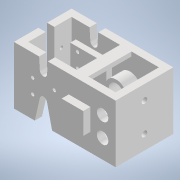
# Autodesk Inventor part: NewCasing
Saved by Autodesk Inventor 2020.1 (Build 241239000, 239)
## iProperties
Created: 2019-11-05
Part Number: NewCasing
Material: Generic
Document SubType Name: Modeling
Designer: ajtan
Density: 1 g/cm^3
Appearance: Default
Author: ajtan
Autodesk Inventor part; units mm, degrees
ref_plane "YZ Plane" through (0, 0, 0) normal (1, 0, 0) x (0, 1, 0)
ref_plane "XZ Plane" through (0, 0, 0) normal (0, 1, 0) x (-1, 0, 0)
ref_plane "XY Plane" through (0, 0, 0) normal (0, 0, 1) x (1, 0, 0)
sketch "Sketch1" plane through (0, 0, 0) normal (0, 0, 1) x (1, 0, 0)
  line L0 (-57.8485, 25.4) -> (-51.4985, 25.4)
  line L1 (-51.4985, 25.4) -> (-51.4985, -25.4)
  line L2 (-51.4985, -25.4) -> (-57.8485, -25.4)
  line L3 (-57.8485, -25.4) -> (-57.8485, 25.4)
  line L4 (25.4, 25.4) -> (31.75, 25.4)
  line L5 (31.75, 25.4) -> (31.75, -25.4)
  line L6 (31.75, -25.4) -> (25.4, -25.4)
  line L7 (25.4, -25.4) -> (25.4, 25.4)
  point P0 (0, 0)
  dimension "d0" = 6.35
  dimension "d1" = 50.8
  dimension "d2" = 25.4
  dimension "d3" = 51.4985
  dimension "d4" = 25.4
  dimension "d5" = 25.4
  constraints: 16 end point, 4 parallel, 2 equal length, 2 horizontal, 2 perpendicular
  measures "d0" distance of L1.end L2.end
  measures "d1" distance of L0.end L1.end
  measures "d2" distance from line of point (0, 0) L0
  measures "d3" distance from line of point (0, 0) L1
  measures "d4" distance from line of point (0, 0) L4
  measures "d5" distance from line of point (0, 0) L7
extrude "Extrusion1" add sketch "Sketch1" along normal mid plane 38.1
sketch "Sketch2" plane through (0, 0, 19.05) normal (0, 0, 1) x (1, 0, 0)
  line L0 (-51.4985, 25.4) -> (-57.8485, 25.4) projected
  line L1 (31.75, -25.4) -> (25.4, -25.4) projected
  line L2 (-57.8485, 25.4) -> (31.75, 25.4)
  line L3 (31.75, 25.4) -> (31.75, -25.4)
  line L4 (31.75, -25.4) -> (-57.8485, -25.4)
  line L5 (-57.8485, -25.4) -> (-57.8485, 25.4)
  circle A0 centre (0, 0) radius 6.604
  circle A1 centre (-41.3385, 6.35) radius 1.4605
  line L6 (-47.9108, 0) -> (-31.2118, 0) construction
  circle A2 centre (-41.3385, -6.35) radius 1.4605
  line L7 (-51.4985, -25.4) -> (-51.4985, 25.4) projected
  dimension "d8" = 13.208
  dimension "d40" = 2.921
  dimension "d42" = 19.05
  dimension "d43" = 16.51
  dimension "d44" = 6.35
  dimension "d92" = 6.35
  constraints: 10 end point, 3 centre point, 2 horizontal, 2 parallel, 1 coincident, 1 perpendicular, 1 symmetric about line, 1 other
  measures "d8" diameter of A0
  measures "d40" diameter of A1
  measures "d42" distance from line of L2 A1.centre
  measures "d43" distance from line of L5 A1.centre
  measures "d44" vertical distance of point (0, 0) A2.centre
  measures "d92" distance between parallel lines of L5 L7
sketch "Sketch3" plane through (0, 0, -19.05) normal (0, 0, -1) x (-1, 0, 0)
  line L0 (-31.75, 25.4) -> (-31.75, -25.4) projected
  line L1 (51.4985, -25.4) -> (57.8485, -25.4) projected
  line L2 (-31.75, 25.4) -> (57.8485, 25.4)
  line L3 (57.8485, 25.4) -> (57.8485, -25.4)
  line L4 (57.8485, -25.4) -> (-31.75, -25.4)
  line L5 (-31.75, -25.4) -> (-31.75, 25.4)
  circle A0 centre (0, 0) radius 6.604
  circle A1 centre (-11.43, 0.0226) radius 2.54
  circle A2 centre (-20.2438, 8.7122) radius 1.7907
  line L6 (-13.9699, 0) -> (6.604, 0) construction
  circle A3 centre (-20.2438, -8.7122) radius 1.7907
  circle A4 centre (41.3385, 6.35) radius 1.4605
  line L7 (51.4985, 25.4) -> (51.4985, -25.4) projected
  circle A5 centre (41.3385, -6.35) radius 1.4605
  dimension "d11" = 13.208
  dimension "d12" = 5.08
  dimension "d13" = 11.43
  dimension "d14" = 3.5814
  dimension "d15" = 20.2438
  dimension "d16" = 8.7122
  dimension "d32" = 2.921
  dimension "d33" = 10.16
  dimension "d34" = 6.35
  dimension "d35" = 6.35
  constraints: 10 end point, 4 centre point, 2 horizontal, 2 parallel, 2 symmetric about line, 1 coincident, 1 horizontal alignment, 1 perpendicular, 7 other
  measures "d13" distance of point (0, 0) point (-11.43, 0.023)
  measures "d14" diameter of A2
  measures "d15" horizontal distance of point (0, 0) A2.centre
  measures "d16" vertical distance of point (0, 0) A2.centre
  measures "d32" diameter of A4
  measures "d33" distance from line of A4.centre L7
  measures "d34" vertical distance of point (0, 0) A4.centre
  measures "d35" vertical distance of point (0, 0) A5.centre
extrude "Extrusion7" add sketch "Sketch2" along normal blind 6.35
extrude "Extrusion6" add sketch "Sketch3" along normal blind 6.35
sketch "Sketch6" plane through (-57.8485, -25.4, 25.4) normal (-1, 0, 0) x (0, 0, 1)
  circle A0 centre (-23.114, 38.1) radius 1.4605
  line L0 (-35.0625, 25.4) -> (-10.5897, 25.4) construction
  line L1 (0, 0) -> (-50.8, 0) construction
  line L2 (0, 50.8) -> (0, 0) construction
  circle A1 centre (-23.114, 12.7) radius 1.4605
  point P0 (-25.4, 25.4)
  dimension "d47" = 2.921
  dimension "d48" = 25.4
  dimension "d49" = 12.7
  dimension "d50" = 23.114
  constraints: 2 centre point, 2 end point, 1 horizontal, 1 symmetric about line, 1 other
  measures "d47" diameter of A0
  measures "d48" distance between parallel lines of L1 L0
  measures "d49" distance from line of L0 A0.centre
  measures "d50" distance from line of L2 A0.centre
extrude "Extrusion8" cut sketch "Sketch6" against normal up to next
sketch "Sketch8" plane through (-57.8485, 25.4, 25.4) normal (0, 1, 0) x (1, 0, 0)
  line L0 (0, 50.8) -> (0, 0) projected
  line L1 (0, 21.59) -> (6.35, 21.59)
  line L2 (6.35, 21.59) -> (6.35, 29.21)
  line L3 (6.35, 29.21) -> (0, 29.21)
  line L4 (0, 29.21) -> (0, 21.59)
  line L5 (0, 25.4) -> (6.35, 25.4) construction
  line L6 (89.5985, 0) -> (0, 0) projected
  line L7 (0, 50.8) -> (89.5985, 50.8) projected
  line L8 (6.35, 6.35) -> (6.35, 44.45) projected
  point P0 (57.8485, 25.4)
  point P1 (0, 29.21)
  dimension "d56" = 25.4
  dimension "d57" = 50.8
  dimension "d58" = 7.62
  constraints: 10 end point, 2 midpoint, 2 parallel, 1 collinear, 1 horizontal, 1 perpendicular, 1 point on line
  measures "d56" distance between parallel lines of L6 L5
  measures "d57" distance between parallel lines of L7 L6
  measures "d58" distance of L1.end L2.end
extrude "Extrusion10" cut sketch "Sketch8" against normal through all
sketch "Sketch10" plane through (0, 0, 25.4) normal (0, 0, 1) x (1, 0, 0)
  circle A0 centre (20.2438, -8.7122) radius 1.7907 construction
  circle A1 centre (20.2438, -8.7122) radius 1.7907 projected
  circle A2 centre (20.2438, 8.7122) radius 1.7907 construction
  circle A3 centre (20.2438, 8.7122) radius 1.7907 projected
  circle A4 centre (20.2438, 8.7122) radius 5.08
  circle A5 centre (20.2438, -8.7122) radius 5.08
  point P0 (0, 0)
  dimension "d64" = 10.16
  constraints: 2 centre point, 2 coincident, 1 equal radius
  measures "d64" diameter of A4
extrude "Extrusion12" cut sketch "Sketch10" against normal blind 25.4 contours A1 | A3 | A4 | A5
sketch "Sketch11" plane through (0, 0, 25.4) normal (0, 0, 1) x (1, 0, 0)
  line L0 (9.525, -9.525) -> (-9.525, -9.525)
  line L1 (-9.525, -9.525) -> (-9.525, 9.525)
  line L2 (-9.525, 9.525) -> (9.525, 9.525)
  line L3 (9.525, 9.525) -> (9.525, -9.525)
  line L4 (9.525, -9.525) -> (-9.525, 9.525) construction
  line L5 (-9.525, -9.525) -> (9.525, 9.525) construction
  point P0 (0, 0)
  dimension "d67" = 19.05
  dimension "d68" = 19.05
  constraints: 12 end point, 2 midpoint, 2 parallel, 1 horizontal, 1 perpendicular
  measures "d67" distance of L1.end L2.end
  measures "d68" distance of L2.end L0.start
extrude "Extrusion13" add sketch "Sketch11" along normal blind 6.35
sketch "Sketch12" plane through (0, 0, -25.4) normal (0, 0, -1) x (-1, 0, 0)
  circle A0 centre (31.8389, -6.35) radius 3.175
  line L0 (57.8485, -25.4) -> (57.8485, 25.4) projected
  line L1 (34.9338, -5.6412) -> (39.4589, -25.4)
  line L2 (28.744, -5.6412) -> (24.2189, -25.4)
  line L3 (24.2189, -25.4) -> (39.4589, -25.4)
  line L4 (-25.4, -25.4) -> (51.4985, -25.4) projected
  circle A1 centre (31.8389, 15.24) radius 3.175
  line L5 (57.8485, 25.4) -> (-31.75, 25.4) projected
  line L6 (28.67, 15.0438) -> (28.0289, 25.4)
  line L7 (51.4985, 25.4) -> (-25.4, 25.4) projected
  line L8 (35.0078, 15.0438) -> (35.6489, 25.4)
  point P0 (0, 0)
  dimension "d71" = 6.35
  dimension "d72" = 26.0096
  dimension "d73" = 6.35
  dimension "d74" = 15.24
  dimension "d75" = 7.62
  dimension "d78" = 10.16
  dimension "d79" = 7.62
  dimension "d80" = 3.81
  constraints: 10 end point, 4 point on circle, 4 tangent, 2 centre point, 2 collinear, 2 point on line, 1 equal radius, 1 vertical alignment
  measures "d71" vertical distance of point (0, 0) A0.centre
  measures "d72" distance from line of L0 A0.centre
  measures "d73" diameter of A0
  measures "d74" distance of L2.end L1.end
  measures "d75" horizontal distance of L2.end A0.centre
  measures "d78" distance from line of L5 A1.centre
  measures "d79" distance of L8.end L6.end
  measures "d80" horizontal distance of A1.centre L6.end
extrude "Extrusion14" cut sketch "Sketch12" against normal through all
sketch "Sketch13" plane through (0, 0, -19.05) normal (0, 0, 1) x (1, 0, 0)
  circle A0 centre (0, 0) radius 6.604 projected
  circle A1 centre (0, 0) radius 6.604 projected
  circle A2 centre (0, 0) radius 9.525
  dimension "d81" = 19.05
  constraints: 1 centre point, 1 coincident
  measures "d81" diameter of A2
extrude "Extrusion15" add sketch "Sketch13" along normal blind 12.192
sketch "Sketch14" plane through (31.75, 25.4, 25.4) normal (0, 1, 0) x (1, 0, 0)
  line L0 (-59.7789, 50.8) -> (0, 50.8) projected
  line L1 (-22.225, 0) -> (-41.275, 0) projected
  line L2 (-40.64, 50.8) -> (-30.48, 50.8)
  line L3 (-30.48, 50.8) -> (-30.48, 0)
  line L4 (-30.48, 0) -> (-40.64, 0)
  line L5 (-40.64, 0) -> (-40.64, 50.8)
  line L6 (0, 0) -> (0, 50.8) projected
  point P0 (-31.75, 25.4)
  dimension "d84" = 10.16
  dimension "d85" = 40.64
  constraints: 8 end point, 2 parallel, 2 point on line, 1 horizontal, 1 perpendicular
  measures "d84" distance between parallel lines of L5 L3
  measures "d85" distance between parallel lines of L6 L5
extrude "Extrusion16" add sketch "Sketch14" against normal blind 3.81
sketch "Sketch15" plane through (0, 0, 19.05) normal (0, 0, -1) x (-1, 0, 0)
  circle A0 centre (0, 0) radius 9.525 projected
  circle A1 centre (0, 0) radius 6.604 projected
extrude "Extrusion17" add sketch "Sketch15" along normal blind 5.08
sketch "Sketch16" plane through (31.75, -25.4, -25.4) normal (0, -1, 0) x (1, 0, 0)
  line L0 (-40.64, 44.45) -> (-30.48, 44.45) projected
  line L1 (-40.64, 44.45) -> (-40.64, 6.35) projected
  line L2 (-30.48, 6.35) -> (-40.64, 6.35) projected
  line L3 (-30.48, 6.35) -> (-30.48, 44.45) projected
  point P0 (-31.75, 25.4)
extrude "Extrusion18" add sketch "Sketch16" against normal blind 3.81
sketch "Sketch17" plane through (0, 0, 25.4) normal (0, 0, 1) x (1, 0, 0)
  arc A0 (-35.0078, 15.0438) -> (-28.67, 15.0438) centre (-31.8389, 15.24) ccw construction
  line L0 (-31.8389, 12.065) -> (-31.8389, -3.175) construction
  arc A1 (-28.744, -5.6412) -> (-34.9338, -5.6412) centre (-31.8389, -6.35) ccw construction
  circle A2 centre (-41.3385, 6.35) radius 1.4605 projected
  circle A3 centre (-41.3385, 6.35) radius 1.4605 projected
  circle A4 centre (-22.3393, 6.35) radius 1.4605
  point P0 (0, 0)
  constraints: 2 end point, 2 point on circle, 1 centre point, 1 symmetric about line, 1 vertical, 1 other
extrude "Extrusion19" cut sketch "Sketch17" against normal through all contours A4
sketch "Sketch19" plane through (-57.8485, -25.4, -25.4) normal (-1, 0, 0) x (0, 0, 1)
  circle A0 centre (15.24, 31.75) radius 1.4605
  circle A1 centre (15.24, 19.05) radius 1.4605
  line L0 (21.59, 0) -> (21.59, 50.8) construction
  line L1 (0, 50.8) -> (21.59, 50.8) construction
  line L2 (25.4, 25.4) -> (25.4, 50.8) construction
  line L3 (6.35, 50.8) -> (44.45, 50.8) construction
  circle A2 centre (35.56, 31.75) radius 1.4605
  circle A3 centre (35.56, 19.05) radius 1.4605
  dimension "d95" = 6.35
  dimension "d96" = 2.921
  dimension "d97" = 2.921
  dimension "d98" = 12.7
  dimension "d99" = 19.05
  constraints: 4 centre point, 2 end point, 2 symmetric about line, 1 midpoint, 1 vertical alignment, 2 other
  measures "d95" distance from line of L0 A0.centre
  measures "d96" diameter of A0
  measures "d97" diameter of A1
  measures "d98" distance of A1.centre A0.centre
  measures "d99" distance from line of L1 A0.centre
extrude "Extrusion20" cut sketch "Sketch19" against normal blind 12.7
sketch "Sketch20" plane through (31.75, -25.4, 25.4) normal (1, 0, 0) x (0, 0, -1)
  circle A0 centre (25.4, 38.1) radius 2.4384
  circle A1 centre (25.4, 12.7) radius 2.4384
  line L0 (50.8, 50.8) -> (50.8, 0) projected
  line L1 (0, 0) -> (0, 50.8) projected
  line L2 (0, 50.8) -> (50.8, 50.8) projected
  point P0 (25.4, 25.4)
  dimension "d102" = 25.4
  dimension "d103" = 50.8
  dimension "d104" = 25.4
  dimension "d105" = 12.7
  dimension "d106" = 4.8768
  constraints: 2 centre point, 1 equal radius, 1 vertical alignment
  measures "d102" distance from line of L0 A0.centre
  measures "d103" distance between parallel lines of L0 L1
  measures "d104" distance of A1.centre A0.centre
  measures "d105" distance from line of L2 A0.centre
  measures "d106" diameter of A0
extrude "Extrusion21" cut sketch "Sketch20" against normal blind 25.4
sketch "Sketch21" plane through (0, 0, -19.05) normal (0, 0, 1) x (1, 0, 0)
  circle A0 centre (-22.3393, 6.35) radius 1.4605 projected
  line L0 (1.27, -21.59) -> (1.27, -25.4) projected
  line L1 (25.4, -25.4) -> (1.27, -25.4) projected
  line L2 (25.4, -25.4) -> (25.4, 25.4) projected
  line L3 (1.27, 25.4) -> (25.4, 25.4) projected
  line L4 (1.27, 25.4) -> (1.27, 21.59) projected
  line L5 (1.27, 21.59) -> (-8.89, 21.59) projected
  line L6 (-8.89, 21.59) -> (-8.89, 25.4) projected
  line L7 (-28.0289, 25.4) -> (-8.89, 25.4) projected
  line L8 (-28.0289, 25.4) -> (-28.67, 15.0438) projected
  arc A1 (-35.0078, 15.0438) -> (-28.67, 15.0438) centre (-31.8389, 15.24) ccw projected
  line L9 (-35.0078, 15.0438) -> (-35.6489, 25.4) projected
  line L10 (-51.4985, 25.4) -> (-35.6489, 25.4) projected
  line L11 (-51.4985, 25.4) -> (-51.4985, -25.4) projected
  line L12 (-39.4589, -25.4) -> (-51.4985, -25.4) projected
  line L13 (-39.4589, -25.4) -> (-34.9338, -5.6412) projected
  arc A2 (-28.744, -5.6412) -> (-34.9338, -5.6412) centre (-31.8389, -6.35) ccw projected
  line L14 (-28.744, -5.6412) -> (-24.2189, -25.4) projected
  line L15 (-8.89, -25.4) -> (-24.2189, -25.4) projected
  line L16 (-8.89, -25.4) -> (-8.89, -21.59) projected
  line L17 (-8.89, -21.59) -> (1.27, -21.59) projected
  circle A3 centre (20.2438, -8.7122) radius 1.7907 projected
  circle A4 centre (20.2438, 8.7122) radius 1.7907 projected
  circle A5 centre (-41.3385, -6.35) radius 1.4605 projected
  circle A6 centre (-41.3385, 6.35) radius 1.4605 projected
  arc A7 (9.3985, 1.5472) -> (9.4045, -1.5101) centre (0, 0) ccw projected
  arc A8 (9.4045, -1.5101) -> (9.3985, 1.5472) centre (11.43, 0.0226) ccw projected
  line L18 (-47.7139, 10.16) -> (-15.9639, 10.16)
  line L19 (-15.9639, 10.16) -> (-15.9639, -10.16)
  line L20 (-15.9639, -10.16) -> (-47.7139, -10.16)
  line L21 (-47.7139, -10.16) -> (-47.7139, 10.16)
  point P0 (-27.7091, -10.16)
  point P1 (-35.9687, -10.16)
  dimension "d109" = 6.3754
  dimension "d110" = 31.75
  dimension "d111" = 20.32
  dimension "d112" = 10.16
  constraints: 8 end point, 2 parallel, 1 horizontal, 1 perpendicular
  measures "d109" distance from line of A6.centre L21
  measures "d110" distance of L18.start L18.end
  measures "d111" distance of L18.end L19.end
  measures "d112" distance from line of point (0, 0) L18
extrude "Extrusion22" add sketch "Sketch21" along normal blind 4.953 contours L14 A2 L13 L20 L21 L18 L19
sketch "Sketch22" plane through (31.75, -25.4, -25.4) normal (0, -1, 0) x (1, 0, 0)
  line L0 (-40.64, 6.35) -> (-40.64, 44.45) projected
  line L1 (-40.64, 18.3213) -> (-30.446, 18.3213)
  line L2 (-30.446, 18.3213) -> (-30.446, 37.9181)
  line L3 (-30.446, 37.9181) -> (-40.64, 37.9181)
  line L4 (-40.64, 37.9181) -> (-40.64, 18.3213)
  point P0 (-31.75, 25.4)
  point P1 (-40.64, 37.9181)
  constraints: 8 end point, 2 parallel, 1 horizontal, 1 perpendicular, 1 point on line
extrude "Extrusion23" cut sketch "Sketch22" against normal blind 6.35
equation "\"d56\" = 0.5 * d57"
equation "\"d75\" = 0.5 * d74"
equation "\"d80\" = 0.5 * d79"
equation "\"d102\" = 0.5 * d103"
equation "\"d107\" = d104"
equation "\"d112\" = 0.5 * d111"
body "Solid1"
